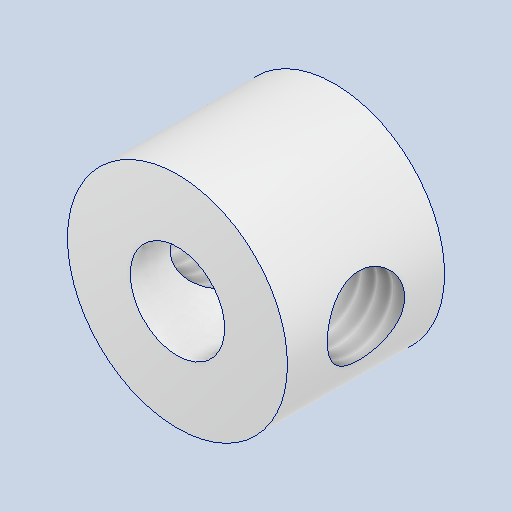
# Autodesk Inventor part: RD014_ストッパ
Saved by Autodesk Inventor 2022 (Build 260153000, 153)
## iProperties
Created: 2021-10-14
Part Number: RD014_ストッパ
Material: アルミニウム 6061
Document SubType Name: Modeling
Designer: gilte
Density: 2.7 g/cm^3
Appearance: アルミニウム - フラット
Author: gilte
Autodesk Inventor part; units mm, degrees
ref_plane "YZ Plane" through (0, 0, 0) normal (1, 0, 0) x (0, 1, 0)
ref_plane "XZ Plane" through (0, 0, 0) normal (0, 1, 0) x (-1, 0, 0)
ref_plane "XY Plane" through (0, 0, 0) normal (0, 0, 1) x (1, 0, 0)
sketch "スケッチ1" plane through (0, 0, 0) normal (0, 0, 1) x (1, 0, 0)
  circle A0 centre (0, 0) radius 3.5
  dimension "d0" = 7
  constraints: 1 centre point, 1 coincident
  measures "d0" diameter of A0
extrude "押し出し1" add sketch "スケッチ1" along normal blind 5
sketch "スケッチ2" plane through (0, 0, 5) normal (0, 0, 1) x (1, 0, 0)
  point P0 (0, 0)
hole "穴1" at (0, 0, 5) direction (0, 0, -1) diameter 3 end through all
sketch "スケッチ3" plane through (0, 0, 0) normal (1, 0, 0) x (0, 1, 0)
  line L0 (1.5, 0) -> (-1.5, 0) projected
  point P0 (0, 0)
  point P1 (0, 2.5)
  dimension "d10" = 2.5
  constraints: 1 vertical alignment
  measures "d10" distance from line of L0 point (0, 2.5)
hole "穴2" at (0, 0, 2.5) direction (-1, 0, 0) diameter 2.459 end through all thread size "M3x0.5" class "6H" standard "ANSI Metric M Profile"
sketch "スケッチ4" plane through (0, 0, 0) normal (1, 0, 0) x (0, 1, 0)
  line L0 (1.5, 0) -> (-1.5, 0) projected
  point P0 (0, 0)
  point P1 (0, 2.5)
  dimension "d18" = 2.5
  constraints: 1 vertical alignment
  measures "d18" distance from line of L0 point (0, 2.5)
hole "穴3" at (0, 0, 2.5) direction (1, 0, 0) diameter 2.459 end through all thread size "M3x0.5" class "6H" standard "ANSI Metric M Profile"
sketch "スケッチ5" plane through (0, 0, 0) normal (1, 0, 0) x (0, 1, 0)
  point P0 (0, 0)
